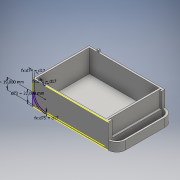
# Autodesk Inventor part: boxMVer1
Saved by Autodesk Inventor 2016 (Build 200138000, 138)
## iProperties
Created: 2015-12-12
Part Number: boxMVer1
Material: Generic
Document SubType Name: Modeling
Designer: hesaon
Density: 1 g/cm^3
Appearance: Default
Author: hesaon
Autodesk Inventor part; units mm, degrees
ref_plane "YZ Plane" through (0, 0, 0) normal (1, 0, 0) x (0, 1, 0)
ref_plane "XZ Plane" through (0, 0, 0) normal (0, 1, 0) x (-1, 0, 0)
ref_plane "XY Plane" through (0, 0, 0) normal (0, 0, 1) x (1, 0, 0)
sketch "Sketch1" plane through (0, 0, 0) normal (0, 0, 1) x (1, 0, 0)
  line L0 (0, 0) -> (132, 0)
  line L1 (0, 0) -> (132, 0)
  line L2 (0, 0) -> (132, 0)
  line L3 (132, 0) -> (132, 99)
  line L4 (132, 99) -> (0, 99)
  line L5 (0, 99) -> (0, 0)
  dimension "d12" = 132
  dimension "d13" = 99
  constraints: 12 end point, 3 horizontal, 2 parallel, 1 perpendicular
  measures "d12" distance of L4.end L3.end
  measures "d13" distance of L3.end L2.end
extrude "Extrusion2" add sketch "Sketch1" along normal blind 3
sketch "Sketch2" plane through (0, 0, 3) normal (0, 0, 1) x (1, 0, 0)
  line L0 (3, 96) -> (125, 96)
  line L1 (125, 96) -> (125, 3)
  line L2 (125, 3) -> (3, 3)
  line L3 (3, 3) -> (3, 96)
  line L4 (132, 99) -> (0, 99) projected
  line L5 (0, 0) -> (132, 0) projected
  line L6 (0, 99) -> (0, 0) projected
  line L7 (132, 0) -> (132, 99) projected
  dimension "d16" = 3
  dimension "d17" = 3
  dimension "d18" = 3
  dimension "d21" = 7
  constraints: 8 end point, 2 parallel, 1 horizontal, 1 perpendicular
  measures "d16" distance from line of L4 L0.start
  measures "d17" distance from line of L5 L2.end
  measures "d18" distance between parallel lines of L6 L3
  measures "d21" distance from line of L7 L1.end
extrude "Extrusion3" add sketch "Sketch2" along normal blind 12
sketch "Sketch3" plane through (0, 0, 0) normal (0, 0, -1) x (-1, 0, 0)
  point P0 (0, 0)
sketch "Sketch4" plane through (0, 0, 0) normal (0, 0, -1) x (-1, 0, 0)
  line L0 (-132, 99) -> (0, 99) projected
  line L1 (-132, 99) -> (-132, 84)
  line L2 (-132, 0) -> (-132, 99) projected
  line L3 (-132, 0) -> (-132, 15)
  arc A0 (-147, 15) -> (-132, 0) centre (-132, 15) ccw
  line L4 (-132, 15) -> (-147, 15) construction
  line L5 (-132, 15) -> (-132, 0) construction
  arc A1 (-132, 99) -> (-147, 84) centre (-132, 84) ccw
  line L6 (-132, 84) -> (-147, 84) construction
  line L7 (-132, 84) -> (-132, 99) construction
  line L8 (-147, 84) -> (-147, 15)
  point P0 (0, 0)
  dimension "d24" = 15
  dimension "d25" = 15
  dimension "d26" = 90
  dimension "d27" = 90
  constraints: 14 end point, 4 point on circle, 2 centre point, 2 coincident, 2 point on line
  measures "d24" distance of L0.start L1.end
  measures "d25" distance of L2.start L3.end
  measures "d26" angle of L4 L5
  measures "d27" angle of L7 L6
extrude "Extrusion4" add sketch "Sketch4" against normal blind 15
sketch "Sketch5" plane through (0, 0, 0) normal (0, 0, -1) x (-1, 0, 0)
  line L0 (-132, 99) -> (0, 99) projected
  line L1 (0, 0) -> (-132, 0) projected
  arc A0 (-132, 95) -> (-144, 83) centre (-132, 83) ccw
  arc A1 (-144, 15) -> (-132, 3) centre (-132, 15) ccw
  line L2 (-144, 83) -> (-144, 15)
  line L3 (-132, 95) -> (-132, 3)
  dimension "d35" = 3
  dimension "d36" = 92
  dimension "d37" = 3
  constraints: 4 end point, 4 point on circle, 2 centre point, 2 vertical
  measures "d35" distance of L1.end L3.end
  measures "d36" distance of L3.start L3.end
extrude "Extrusion5" cut sketch "Sketch5" against normal through all
sketch "Sketch6" plane through (0, 0, 15) normal (0, 0, 1) x (1, 0, 0)
  line L0 (132, 99) -> (0, 99) projected
  arc A0 (147, 84) -> (132, 99) centre (132, 84) ccw projected
  line L1 (0, 99) -> (132, 99)
  line L2 (132, 99) -> (132, 93)
  line L3 (132, 3) -> (132, 95) projected
  line L4 (132, 93) -> (129, 93)
  line L5 (129, 93) -> (129, 96)
  line L6 (129, 96) -> (128, 96)
  line L7 (128, 96) -> (128, 4)
  line L8 (125, 96) -> (125, 3) projected
  line L9 (128, 4) -> (129, 4)
  line L10 (129, 4) -> (129, 7)
  line L11 (129, 7) -> (132, 7)
  line L12 (132, 7) -> (132, 0)
  line L13 (0, 0) -> (132, 0) projected
  line L14 (132, 0) -> (0, 0)
  line L15 (0, 99) -> (0, 0) projected
  line L16 (0, 0) -> (0, 99)
  line L17 (3, 96) -> (125, 96) projected
  line L18 (3, 96) -> (125, 96)
  line L19 (125, 96) -> (125, 3)
  line L20 (125, 3) -> (3, 3)
  line L21 (3, 3) -> (3, 96)
  dimension "d40" = 6
  dimension "d41" = 3
  dimension "d42" = 3
  dimension "d43" = 1
  dimension "d44" = 3
  dimension "d45" = 3
  constraints: 32 end point, 6 perpendicular, 4 point on line, 3 collinear, 3 parallel, 1 horizontal, 1 tangent
  measures "d40" distance of L0.start L2.end
  measures "d41" distance of L2.end L4.end
  measures "d42" distance of L4.end L5.end
  measures "d43" distance of L5.end L6.end
  measures "d44" distance of L9.end L10.end
  measures "d45" distance of L10.end L11.end
extrude "Extrusion6" add sketch "Sketch6" along normal blind 27.5 contours L2 L4 L5 L6 L7 L9 L10 L11 L3 L12 L13 L15 L0
sketch "Sketch7" plane through (0, 0, 42.5) normal (0, 0, 1) x (1, 0, 0)
  line L0 (0, 99) -> (0, 0) projected
  line L1 (0, 0) -> (16, 0)
  line L2 (0, 0) -> (132, 0) projected
  line L3 (3, 3) -> (125, 3) projected
  line L4 (16, 0) -> (19, 0)
  line L5 (19, 0) -> (19, 3)
  line L6 (19, 3) -> (16, 3)
  line L7 (16, 3) -> (16, 0)
  line L8 (0, 99) -> (16, 99)
  line L9 (132, 99) -> (0, 99) projected
  line L10 (125, 96) -> (3, 96) projected
  line L11 (16, 99) -> (19, 99)
  line L12 (19, 99) -> (19, 96)
  line L13 (19, 96) -> (16, 96)
  line L14 (16, 96) -> (16, 99)
  dimension "d48" = 16
  dimension "d49" = 3
  dimension "d50" = 16
  dimension "d51" = 3
  constraints: 20 end point, 4 parallel, 4 point on line, 2 horizontal, 2 perpendicular
  measures "d48" distance of L0.end L1.end
  measures "d49" distance of L6.end L5.end
  measures "d50" distance of L0.start L8.end
  measures "d51" distance of L12.end L13.end
extrude "Extrusion7" add sketch "Sketch7" along normal blind 4
sketch "Sketch10" plane through (0, 0, 0) normal (0, -1, 0) x (1, 0, 0)
  line L0 (132, 42.5) -> (19, 42.5) projected
  line L1 (19, 42.5) -> (22, 42.5)
  line L2 (22, 3) -> (22, 0)
  line L3 (0, 0) -> (132, 0) projected
  line L4 (0, 0) -> (0, 22)
  line L5 (0, 0) -> (0, 42.5) projected
  line L6 (0, 22) -> (3, 22)
  arc A0 (0, 22) -> (22, 0) centre (22, 22) ccw
  line L7 (125, 3) -> (3, 3) projected
  arc A1 (3, 22) -> (22, 3) centre (22, 22) ccw
  line L8 (19, 3.2383) -> (19, 3)
  line L9 (19, 0.2055) -> (19, 0)
  dimension "d70" = 3
  dimension "d73" = 22
  dimension "d74" = 3
  dimension "d75" = 3
  dimension "d76" = 19
  constraints: 12 end point, 6 point on circle, 5 point on line, 2 centre point, 2 vertical, 1 coincident, 1 horizontal, 1 perpendicular
  measures "d70" distance of L0.end L1.end
  measures "d73" distance from line of L3 L6.end
  measures "d74" distance of L6.end L4.end
  measures "d75" distance of L2.end L2.start
  measures "d76" distance of A0.centre L2.start
equation "\"d16\" = d17"
equation "\"d18\" = d17"
equation "\"d25\" = d24"
equation "\"d35\" = d17"
equation "\"d37\" = d17"
equation "\"d41\" = d17"
equation "\"d42\" = d17"
equation "\"d44\" = d17"
equation "\"d45\" = d17"
equation "\"d49\" = d17"
equation "\"d51\" = d17"
equation "\"d70\" = d17"
equation "\"d74\" = d17"
equation "\"d75\" = d17"
body "Solid2"
